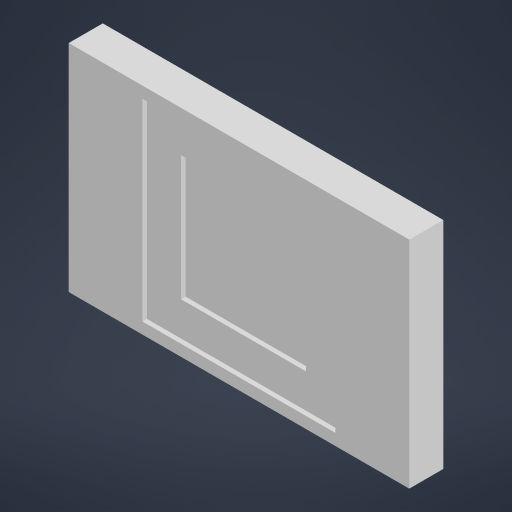
# Autodesk Inventor part: Shoulder_Both_Marker_V1
Saved by Autodesk Inventor 2024 (Build 280153000, 153)
## iProperties
Created: 2023-07-12
Part Number: Shoulder_Both_Marker_V1
Material: Generic
Document SubType Name: Modeling
Designer: User
Density: 1 g/cm^3
Appearance: Default
Author: User
Autodesk Inventor part; units mm, degrees
ref_plane "YZ Plane" through (0, 0, 0) normal (1, 0, 0) x (0, 1, 0)
ref_plane "XZ Plane" through (0, 0, 0) normal (0, 1, 0) x (-1, 0, 0)
ref_plane "XY Plane" through (0, 0, 0) normal (0, 0, 1) x (1, 0, 0)
sketch "Sketch1" plane through (0, 0, 0) normal (0, 0, 1) x (1, 0, 0)
  line L0 (0, 0) -> (-150, 0)
  line L1 (-150, 0) -> (-150, 95)
  line L2 (-150, 95) -> (0, 95)
  line L3 (0, 95) -> (0, 0)
  dimension "d0" = 150
  dimension "d1" = 95
  constraints: 8 end point, 2 parallel, 1 horizontal, 1 perpendicular
  measures "d0" distance of L1.end L2.end
  measures "d1" distance of L0.end L1.end
extrude "Extrusion1" add sketch "Sketch1" along normal blind 15
sketch "Sketch2" plane through (0, 0, 15) normal (0, 0, 1) x (1, 0, 0)
  line L0 (-32.5, 5) -> (-117.5, 5)
  line L1 (-117.5, 5) -> (-117.5, 90)
  line L2 (-117.5, 90) -> (-32.5, 90)
  line L3 (-32.5, 90) -> (-32.5, 5)
  point P0 (0, 0)
  dimension "d4" = 85
  dimension "d5" = 85
  constraints: 8 end point, 2 parallel, 1 horizontal, 1 perpendicular, 1 other
  measures "d4" distance of L1.end L2.end
  measures "d5" distance of L0.end L1.end
extrude "Extrusion2" cut sketch "Sketch2" against normal blind 2
sketch "Sketch3" plane through (0, 0, 13) normal (0, 0, 1) x (1, 0, 0)
  line L0 (-47.5, 75) -> (-102.5, 75)
  line L1 (-102.5, 75) -> (-102.5, 20)
  line L2 (-102.5, 20) -> (-47.5, 20)
  line L3 (-47.5, 20) -> (-47.5, 75)
  point P0 (0, 0)
  point P1 (-47.5, 47.5)
  dimension "d10" = 55
  dimension "d11" = 55
  constraints: 8 end point, 2 parallel, 1 horizontal, 1 perpendicular, 1 other
  measures "d10" distance of L2.end L1.end
  measures "d11" distance of L1.end L0.end
extrude "Extrusion3" cut sketch "Sketch3" against normal blind 2
sketch "Sketch4" plane through (0, 0, 0) normal (0, 0, -1) x (-1, 0, 0)
  circle A0 centre (75, 47.5) radius 14.25
  circle A1 centre (75, 47.5) radius 17.15
  line L0 (2.5, 2.5) -> (7.5, 2.5)
  line L1 (7.5, 2.5) -> (7.5, 7.5)
  line L2 (7.5, 7.5) -> (2.5, 7.5)
  line L3 (2.5, 7.5) -> (2.5, 2.5)
  line L4 (147.5, 2.5) -> (142.5, 2.5)
  line L5 (142.5, 2.5) -> (142.5, 7.5)
  line L6 (142.5, 7.5) -> (147.5, 7.5)
  line L7 (147.5, 7.5) -> (147.5, 2.5)
  line L8 (2.5, 92.5) -> (7.5, 92.5)
  line L9 (7.5, 92.5) -> (7.5, 87.5)
  line L10 (7.5, 87.5) -> (2.5, 87.5)
  line L11 (2.5, 87.5) -> (2.5, 92.5)
  line L12 (147.5, 92.5) -> (142.5, 92.5)
  line L13 (142.5, 92.5) -> (142.5, 87.5)
  line L14 (142.5, 87.5) -> (147.5, 87.5)
  line L15 (147.5, 87.5) -> (147.5, 92.5)
  point P0 (0, 0)
  dimension "d14" = 28.5
  dimension "d15" = 34.3
  dimension "d16" = 5
  dimension "d17" = 5
  dimension "d18" = 5
  dimension "d19" = 5
  dimension "d20" = 5
  dimension "d21" = 5
  dimension "d22" = 5
  dimension "d23" = 5
  constraints: 32 end point, 8 parallel, 4 horizontal, 4 perpendicular, 2 centre point, 2 coincident
  measures "d14" diameter of A0
  measures "d15" diameter of A1
  measures "d16" distance of L2.end L1.end
  measures "d17" distance of L1.end L0.end
  measures "d18" distance of L5.end L6.end
  measures "d19" distance of L4.end L5.end
  measures "d20" distance of L9.end L10.end
  measures "d21" distance of L8.end L9.end
  measures "d22" distance of L14.end L13.end
  measures "d23" distance of L13.end L12.end
extrude "Extrusion4" cut sketch "Sketch4" against normal blind 5
body "Solid1"
